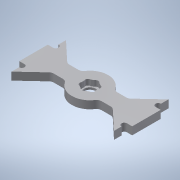
# Autodesk Inventor part: 足首_サブフレーム_1_3
Saved by Autodesk Inventor 2020 (Build 240168000, 168)
## iProperties
Created: 2016-04-30
Part Number: 足首_サブフレーム_1_3
Material: アルミニウム 2014-T4
Document SubType Name: Modeling
Designer: hiroaki
Density: 2.8 g/cm^3
Appearance: サテン
Mass: 4.12738 g
Surface Area: 15.3831 cm^2
Volume: 1.47406 cm^3
Category: 足首
Author: hiroaki
Autodesk Inventor part; units mm, degrees
ref_plane "YZ Plane" through (0, 0, 0) normal (1, 0, 0) x (0, 1, 0)
ref_plane "XZ Plane" through (0, 0, 0) normal (0, 1, 0) x (-1, 0, 0)
ref_plane "XY Plane" through (0, 0, 0) normal (0, 0, 1) x (1, 0, 0)
sketch "スケッチ1" plane through (0, 0, 0) normal (0, 0, 1) x (1, 0, 0)
  line L0 (-21.75, 5.5) -> (-21.75, -5.5)
  line L1 (-21.75, -5.5) -> (-19.75, -5.5)
  line L2 (-21.75, 5.5) -> (-19.75, 5.5)
  line L3 (-19.75, 7.6) -> (-19.75, 10.5)
  line L4 (-19.75, 10.5) -> (19.75, 10.5)
  line L5 (19.75, 10.5) -> (19.75, 7.6)
  line L6 (-19.75, -7.6) -> (-19.75, -10.5)
  line L7 (-19.75, -10.5) -> (19.75, -10.5)
  line L8 (19.75, -10.5) -> (19.75, -7.6)
  line L9 (19.75, 5.5) -> (21.75, 5.5)
  line L10 (21.75, 5.5) -> (21.75, -5.5)
  line L11 (21.75, -5.5) -> (19.75, -5.5)
  line L12 (0, 0) -> (0, 10.5) construction
  line L13 (0, 0) -> (-21.75, 0) construction
  arc A0 (-19.75, 5.5) -> (-19.75, 7.6) centre (-19.75, 6.55) ccw
  arc A1 (-19.75, -7.6) -> (-19.75, -5.5) centre (-19.75, -6.55) ccw
  arc A2 (19.75, 7.6) -> (19.75, 5.5) centre (19.75, 6.55) ccw
  arc A3 (19.75, -5.5) -> (19.75, -7.6) centre (19.75, -6.55) ccw
  circle A4 centre (0, 0) radius 2.25
  dimension "d0" = 39.5
  dimension "d1" = 2
  dimension "d2" = 11
  dimension "d8" = 1.05
  dimension "d10" = 5
  dimension "d12" = 4.5
  constraints: 28 end point, 9 perpendicular, 8 point on circle, 5 centre point, 4 symmetric about line, 4 vertical alignment, 3 tangent, 3 vertical, 2 equal radius, 2 horizontal, 2 midpoint, 1 coincident, 2 other
  measures "d0" distance of L3.end L4.end
  measures "d1" distance between parallel lines of L0 L3
  measures "d2" distance of L0.start L0.end
  measures "d8" radius of A0
  measures "d10" distance between parallel lines of L2 L4
  measures "d12" diameter of A4
extrude "押し出し1" add sketch "スケッチ1" along normal blind 3
sketch "スケッチ2" plane through (0, 0, 0) normal (0, 0, -1) x (-1, 0, 0)
  circle A0 centre (0, 0) radius 2.25 projected
  line L0 (-19.75, 10.5) -> (19.75, 10.5) projected
  line L1 (-21.75, -5.5) -> (-21.75, 5.5) projected
  arc A1 (6.3246, 3) -> (-6.3246, 3) centre (0, 0) ccw
  line L2 (-6.3246, 3) -> (-11.75, 3)
  line L3 (-11.75, 3) -> (-23.9536, 14.4408)
  line L4 (-23.9536, 14.4408) -> (23.9536, 14.4408)
  line L5 (23.9536, 14.4408) -> (11.75, 3)
  line L6 (11.75, 3) -> (6.3246, 3)
  line L7 (-19.75, 10.5) -> (19.75, 10.5) construction
  line L8 (0, 10.5) -> (0, 0) construction
  line L9 (0, 0) -> (-21.75, 0) construction
  arc A2 (-6.3246, -3) -> (6.3246, -3) centre (0, 0) ccw
  line L10 (-6.3246, -3) -> (-11.75, -3)
  line L11 (-11.75, -3) -> (-23.9536, -14.4408)
  line L12 (-23.9536, -14.4408) -> (23.9536, -14.4408)
  line L13 (23.9536, -14.4408) -> (11.75, -3)
  line L14 (11.75, -3) -> (6.3246, -3)
  dimension "d17" = 7
  dimension "d19" = 3
  dimension "d38" = 8
  constraints: 24 end point, 7 symmetric about line, 4 point on circle, 2 centre point, 2 midpoint, 2 point on line, 1 coincident, 1 collinear, 1 horizontal, 1 horizontal alignment, 1 parallel, 1 vertical, 1 other
  measures "d17" radius of A1
  measures "d19" distance from line of A0.centre L2
  measures "d38" horizontal distance of L0.start L2.end
extrude "押し出し2" cut sketch "スケッチ2" against normal blind 10 contours L3 L4 L5 L0 | L0 L5 L6 A1 L2 L3 | A2 L14 L13 L12 L11 L10
fillet "フィレット1" radius 2 8 edges at (6.3246, 3, 1.5) (-6.3246, 3, 1.5) (6.3246, -3, 1.5) (-6.3246, -3, 1.5) (11.75, -3, 1.5) (11.75, 3, 1.5) (-11.75, 3, 1.5) (-11.75, -3, 1.5)
sketch "スケッチ3" plane through (0, 0, 3) normal (0, 0, 1) x (1, 0, 0)
  circle A0 centre (0, 0) radius 2.25 projected
  line L0 (2.75, 1.5877) -> (2.75, -1.5877)
  line L1 (2.75, -1.5877) -> (0, -3.1754)
  line L2 (0, -3.1754) -> (-2.75, -1.5877)
  line L3 (-2.75, -1.5877) -> (-2.75, 1.5877)
  line L4 (-2.75, 1.5877) -> (0, 3.1754)
  line L5 (0, 3.1754) -> (2.75, 1.5877)
  line L6 (0, 3.187) -> (-2.76, 1.5935)
  line L7 (-2.76, 1.5935) -> (-2.76, -1.5935)
  line L8 (-2.76, -1.5935) -> (0, -3.187)
  line L9 (0, -3.187) -> (2.76, -1.5935)
  line L10 (2.76, -1.5935) -> (2.76, 1.5935)
  line L11 (2.76, 1.5935) -> (0, 3.187)
  circle A1 centre (0, 2.137) radius 1.05
  circle A2 centre (-1.8507, 1.0685) radius 1.05
  circle A3 centre (-1.8507, -1.0685) radius 1.05
  circle A4 centre (0, -2.137) radius 1.05
  circle A5 centre (1.8507, -1.0685) radius 1.05
  circle A6 centre (1.8507, 1.0685) radius 1.05
  point P0 (-2.76, 1.5935)
  point P1 (-2.76, -1.5935)
  point P2 (0, -3.187)
  point P3 (2.76, -1.5935)
  point P4 (2.76, 1.5935)
  dimension "d47" = 2.1
  dimension "d46" = 5.5
  dimension "d48" = 0.01
  dimension "d51" = 360
  constraints: 24 end point, 3 vertical alignment, 1 coincident, 1 vertical, 53 other
  measures "d46" distance between parallel lines of L0 L3
  measures "d48" distance between parallel lines of L6 L4
extrude "押し出し3" cut sketch "スケッチ3" against normal blind 2.2 contours A0 A6 L0 A5 | A6 A0 | A0 A6 L5 L0 | A5 L0 L1 A0 | A0 A5 | A0 A1 L5 A6 | A6 L10 A5 L0 | L0 L5 A6 L11 L10 | A5 L1 A4 A0 | A5 L10 L9 L1 L0 | A1 A0 | A0 A1 L4 L5 | L5 A1 L11 A6 | L10 A6 | A4 L1 L2 A0 | A0 A4 | A5 L9 A4 L1 | A5 L10 | A0 A2 L4 A1 | L5 L4 A1 L6 L11 | A6 L11 | A4 L2 A3 A0 | A4 L9 L8 L2 L1 | L9 A5 | A2 A0 | A0 A2 L3 L4 | L4 A2 L6 A1 | L11 A1 | A3 L2 L3 A0 | A0 A3 | A4 L8 A3 L2 | A4 L9 | A0 A3 L3 A2 | L4 L3 A2 L7 L6 | A1 L6 | A3 L8 L7 L3 L2 | L8 A4 | L3 A3 L7 A2 | L6 A2 | A3 L8 | A2 L7 | L7 A3
equation "\"d2\" = d3"
equation "\"d10\" = d27"
equation "\"d3\" = 11"
equation "\"d27\" = 5"
